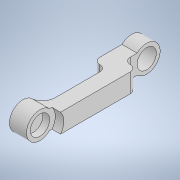
# Autodesk Inventor part: Рулевая тяга
Saved by Autodesk Inventor 2020 (Build 240168000, 168)
## iProperties
Created: 2021-07-18
Part Number: Рулевая тяга
Material: Типовые
Document SubType Name: Modeling
Designer: Антон
Density: 1 g/cm^3
Appearance: По умолчанию
Author: Антон
Autodesk Inventor part; units mm, degrees
ref_plane "YZ Plane" through (0, 0, 0) normal (1, 0, 0) x (0, 1, 0)
ref_plane "XZ Plane" through (0, 0, 0) normal (0, 1, 0) x (-1, 0, 0)
ref_plane "XY Plane" through (0, 0, 0) normal (0, 0, 1) x (1, 0, 0)
sketch "Эскиз1" plane through (0, 0, 0) normal (0, 1, 0) x (-1, 0, 0)
  line L0 (0, 0) -> (4, 0)
  line L1 (4, 0) -> (4, -23.1503)
  line L2 (4, -23.1503) -> (0, -23.1503)
  line L3 (0, -23.1503) -> (0, 0)
  line L4 (0, -23.1503) -> (7.35, -23.1503)
  line L5 (7.35, -23.1503) -> (7.35, -19.1503)
  line L6 (7.35, -19.1503) -> (0, -19.1503)
  line L7 (0, -19.1503) -> (0, -23.1503)
  line L8 (7.35, -19.1503) -> (3.35, -19.1503)
  line L9 (3.35, -19.1503) -> (3.35, -29.1503)
  line L10 (3.35, -29.1503) -> (7.35, -29.1503)
  line L11 (7.35, -29.1503) -> (7.35, -19.1503)
  line L12 (7.35, -23.1503) -> (4, -19.1503)
  line L13 (0, -19.1503) -> (3.35, -23.1503)
  point P0 (4, -19.1503)
  point P1 (0, -19.1503)
  point P2 (4, -19.1503)
  dimension "d10" = 4
  dimension "d11" = 7.35
  dimension "d36" = 29.1503
  dimension "d57" = 10
  constraints: 28 end point, 6 parallel, 4 point on line, 3 horizontal, 3 perpendicular, 2 equal length
  measures "d10" distance of L0.start L0.end
  measures "d11" distance between parallel lines of L3 L11
  measures "d36" distance between parallel lines of L10 L0
  measures "d57" distance of L10.end L5.end
extrude "Выдавливание1" add sketch "Эскиз1" along normal blind 5
fillet "Сопряжение2" radius 1.675 4 edges at (-4, 2.5, -19.1503) (-7.35, 2.5, -19.1503) (-3.35, 2.5, -23.1503) (0, 2.5, -23.1503)
sketch "Эскиз7" plane through (-7.35, 0, -29.1503) normal (-1, 0, 0) x (0, 0, 1)
  line L0 (0, 0) -> (0, 5) projected
  circle A0 centre (0, 2.5) radius 2.525
  circle A1 centre (0, 2.5) radius 3.525
  point P0 (29.1503, 0)
  point P1 (0, 4.975)
  point P2 (0, 0.025)
  dimension "d37" = 5.05
  dimension "d38" = 7.05
  constraints: 2 centre point, 1 coincident, 1 midpoint
  measures "d37" diameter of A0
  measures "d38" diameter of A1
extrude "Выдавливание5" add sketch "Эскиз7" against normal up to surface (4 mm away) contours A0 | A1
extrude "Выдавливание8" cut sketch "Эскиз7" against normal through all contours A0
sketch "Эскиз8" plane through (-4, 0, 0) normal (-1, 0, 0) x (0, 0, 1)
  line L0 (0, 0) -> (0, 5) projected
  circle A0 centre (0, 2.5) radius 2.525
  circle A1 centre (0, 2.5) radius 3.525
  point P0 (0, 4.975)
  point P1 (0, 0.025)
  dimension "d41" = 5.05
  dimension "d42" = 7.05
  constraints: 2 centre point, 1 coincident, 1 midpoint
  measures "d41" diameter of A0
  measures "d42" diameter of A1
extrude "Выдавливание6" add sketch "Эскиз8" against normal up to surface (4 mm away)
extrude "Выдавливание7" cut sketch "Эскиз8" against normal through all contours A0
sketch "Эскиз13" plane through (0, 0, -21.4753) normal (1, 0, 0) x (0, 0, -1)
  arc A0 (-18.9902, 5) -> (-18.9902, 0) centre (-21.4753, 2.5) ccw projected
  circle A1 centre (-21.4753, 2.5) radius 4.025
  point P0 (-21.4753, 0)
  dimension "d66" = 0.5
  constraints: 1 centre point, 1 coincident
  measures "d66" radial gap between concentric circles of A0 A1
extrude "Выдавливание13" cut sketch "Эскиз13" against normal blind 2.25
sketch "Эскиз10" plane through (-4, 0, -17.4753) normal (-1, 0, 0) x (0, 0, 1)
  circle A0 centre (17.4753, 2.5) radius 2.525 projected
  circle A1 centre (17.4753, 2.5) radius 3.525
  arc A2 (14.9902, 0) -> (14.9902, 5) centre (17.4753, 2.5) ccw projected
  constraints: 1 centre point, 1 coincident, 1 concentric
extrude "Выдавливание10" add sketch "Эскиз10" along normal blind 2.25 contours A0 | A1
sketch "Эскиз11" plane through (-6.25, 2.5, 0) normal (-1, 0, 0) x (0, 0, 1)
  circle A0 centre (0, 0) radius 3.525 projected
  point P0 (0, -2.5)
extrude "Выдавливание11" add sketch "Эскиз11" along normal blind 0.5
fillet "Сопряжение6" radius 2.75 1 edges at (-4, 2.5, -3.525)
sketch "Эскиз12" plane through (-4, 0, -17.4753) normal (-1, 0, 0) x (0, 0, 1)
  line L0 (6.7198, 0) -> (2.7198, 0) construction
  line L1 (6.7198, 1) -> (2.7198, 1)
  line L2 (2.7198, -1) -> (6.7198, -1)
  arc A0 (6.7198, -1) -> (6.7198, 1) centre (6.7198, 0) ccw
  arc A1 (2.7198, 1) -> (2.7198, -1) centre (2.7198, 0) ccw
  line L3 (0, 0) -> (11.7198, 0) projected
  point P0 (17.4753, 0)
  point P1 (4.7198, 0)
  dimension "d58" = 2
  dimension "d59" = 2
  dimension "d63" = 7
  constraints: 8 end point, 4 point on circle, 4 tangent, 2 centre point, 1 collinear, 1 horizontal, 1 midpoint, 1 parallel
  measures "d58" distance of point (4.72, 0) L0.end
  measures "d59" diameter of A1
  measures "d63" distance of L3.end point (4.72, 0)
extrude "Выдавливание12" cut sketch "Эскиз12" against normal blind 1.55
